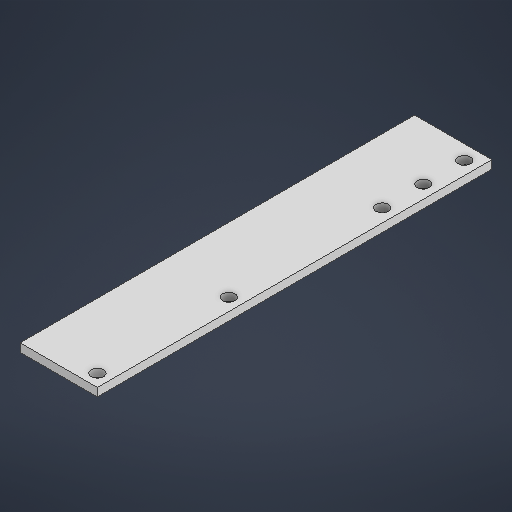
# Autodesk Inventor part: connectStepper
Saved by Autodesk Inventor 2026.2 (Build 302298000, 298)
## iProperties
Created: 2026-04-06
Part Number: connectStepper
Material: Generic
Document SubType Name: Modeling
Designer: Brian Wang
Density: 1 g/cm^3
Appearance: Default
Author: Brian Wang
Autodesk Inventor part; units mm, degrees
ref_plane "YZ Plane" through (0, 0, 0) normal (1, 0, 0) x (0, 1, 0)
ref_plane "XZ Plane" through (0, 0, 0) normal (0, 1, 0) x (-1, 0, 0)
ref_plane "XY Plane" through (0, 0, 0) normal (0, 0, 1) x (1, 0, 0)
sketch "Sketch1" plane through (0, 0, 0) normal (0, 1, 0) x (-1, 0, 0)
  line L0 (12.3827, 15.7347) -> (-6.4173, 15.7347)
  line L1 (-6.4173, 15.7347) -> (-6.4173, -80.2653)
  line L2 (-6.4173, -80.2653) -> (12.3827, -80.2653)
  line L3 (12.3827, -80.2653) -> (12.3827, 15.7347)
  circle A0 centre (-3.4173, 12.7347) radius 1.5
  circle A1 centre (-3.4173, -19.2653) radius 1.5
  circle A2 centre (-3.2173, -76.7547) radius 1.5
  circle A3 centre (-3.2173, -66.7547) radius 1.5
  circle A4 centre (-3.2173, -56.7547) radius 1.5
  point P0 (0, 0)
  dimension "d0" = 3
  dimension "d1" = 18.8
  dimension "d2" = 96
  dimension "d3" = 3
  dimension "d4" = 32
  dimension "d5" = 35
  dimension "d6" = 3
  dimension "d7" = 3
  dimension "d8" = 3
  dimension "d9" = 3
  dimension "d10" = 3
  dimension "d11" = 10
  dimension "d12" = 10
  dimension "d13" = 3.2
  constraints: 8 end point, 5 centre point, 2 parallel, 1 horizontal, 1 perpendicular
  measures "d0" diameter of A0
  measures "d1" distance of L0.start L0.end
  measures "d2" distance of L2.end L0.start
  measures "d3" diameter of A1
  measures "d4" distance of A0.centre A1.centre
  measures "d5" distance from line of L0 A1.centre
  measures "d6" distance from line of L1 A0.centre
  measures "d7" distance from line of L1 A1.centre
  measures "d8" diameter of A2
  measures "d9" diameter of A3
  measures "d10" diameter of A4
  measures "d11" distance of A3.centre A2.centre
  measures "d12" distance of A4.centre A3.centre
  measures "d13" distance from line of L1 A4.centre
extrude "Extrusion1" add sketch "Sketch1" along normal blind 2
body "Solid1"
